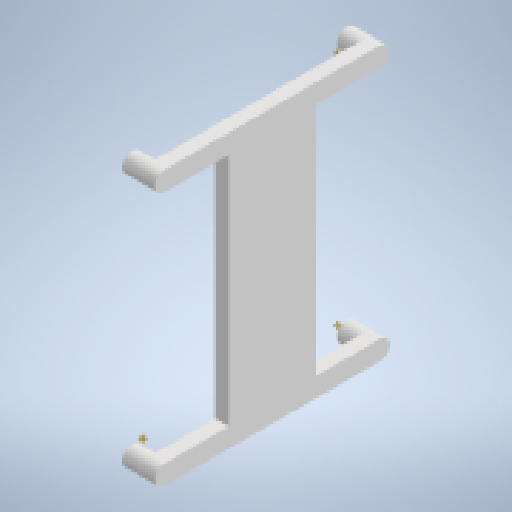
# Autodesk Inventor part: base
Saved by Autodesk Inventor 2025.2 (Build 292293000, 293)
## iProperties
Created: 2025-02-22
Part Number: base
Material: Générique
Document SubType Name: Modeling
Designer: antoi
Density: 1 g/cm^3
Appearance: Par défaut
Author: antoi
Autodesk Inventor part; units mm, degrees
ref_plane "YZ Plane" through (0, 0, 0) normal (1, 0, 0) x (0, 1, 0)
ref_plane "XZ Plane" through (0, 0, 0) normal (0, 1, 0) x (-1, 0, 0)
ref_plane "XY Plane" through (0, 0, 0) normal (0, 0, 1) x (1, 0, 0)
sketch "Esquisse1" plane through (0, 0, 0) normal (1, 0, 0) x (0, 1, 0)
  line L0 (7.5, 0) -> (138.9, 0)
  line L1 (146.4, -7.5) -> (146.4, -122.5)
  line L2 (138.9, -130) -> (7.5, -130)
  line L3 (0, -122.5) -> (0, -7.5)
  arc A0 (138.9, -130) -> (146.4, -122.5) centre (138.9, -122.5) ccw
  arc A1 (0, -122.5) -> (7.5, -130) centre (7.5, -122.5) ccw
  arc A2 (7.5, 0) -> (0, -7.5) centre (7.5, -7.5) ccw
  arc A3 (146.4, -7.5) -> (138.9, 0) centre (138.9, -7.5) ccw
  line L4 (15, -42.5) -> (131.4, -42.5)
  line L5 (131.4, -42.5) -> (131.4, -87.5)
  line L6 (131.4, -87.5) -> (15, -87.5)
  line L7 (15, -87.5) -> (15, -42.5)
  circle A4 centre (138.9, -122.5) radius 7.5
  line L8 (15, -42.5) -> (15, 0)
  line L9 (15, -87.5) -> (15, -130)
  line L10 (131.4, -87.5) -> (131.4, -130)
  line L11 (131.4, -42.5) -> (131.4, 0)
  circle A5 centre (7.5, -122.5) radius 7.5
  circle A6 centre (138.9, -7.5) radius 7.5
  circle A7 centre (7.5, -7.5) radius 7.5
  point P0 (0, 0)
  point P1 (146.4, -130)
  point P2 (146.4, 0)
  point P3 (0, -130)
  point P4 (73.2, -87.5)
  dimension "d0" = 146.4
  dimension "d1" = 130
  dimension "d2" = 7.5
  dimension "d3" = 7.5
  dimension "d4" = 116.4
  dimension "d5" = 45
  dimension "d11" = 42.5
  dimension "d12" = 42.5
  dimension "d13" = 15
  dimension "d104" = 131.4
  dimension "d107" = 115
  constraints: 24 end point, 14 point on line, 8 centre point, 8 point on circle, 8 tangent, 4 parallel, 4 perpendicular, 3 equal radius, 3 horizontal, 1 coincident, 1 midpoint, 1 vertical, 6 other
  measures "d0" distance of point (146.4, -130) point (0, -130)
  measures "d1" distance of point (146.4, 0) point (146.4, -130)
  measures "d2" radius of A0
  measures "d3" radius of A1
  measures "d4" distance of L5.end L6.end
  measures "d5" distance of L4.end L5.end
  measures "d11" distance between parallel lines of L0 L4
  measures "d12" distance from line of L2 point (73.2, -87.5)
  measures "d13" distance between parallel lines of L1 L10
  measures "d104" distance of A4.centre A5.centre
  measures "d107" distance of A4.centre A6.centre
sketch "Esquisse1 outline for Extrusion1" plane through (0, 0, 0) normal (1, 0, 0) x (0, 1, 0)
  line L0 (15, -87.5) -> (131.4, -87.5)
  line L1 (15, -130) -> (15, -87.5)
  line L2 (7.5, -130) -> (15, -130)
  arc A0 (0, -122.5) -> (7.5, -130) centre (7.5, -122.5) ccw
  line L3 (0, -7.5) -> (0, -122.5)
  arc A1 (7.5, 0) -> (0, -7.5) centre (7.5, -7.5) ccw
  line L4 (15, 0) -> (7.5, 0)
  line L5 (15, -42.5) -> (15, 0)
  line L6 (131.4, -42.5) -> (15, -42.5)
  line L7 (131.4, 0) -> (131.4, -42.5)
  line L8 (138.9, 0) -> (131.4, 0)
  arc A2 (146.4, -7.5) -> (138.9, 0) centre (138.9, -7.5) ccw
  line L9 (146.4, -122.5) -> (146.4, -7.5)
  arc A3 (138.9, -130) -> (146.4, -122.5) centre (138.9, -122.5) ccw
  line L10 (131.4, -130) -> (138.9, -130)
  line L11 (131.4, -87.5) -> (131.4, -130)
extrude "Extrusion1" add sketch "Esquisse1 outline for Extrusion1" along normal blind 7
sketch "Esquisse2" plane through (0, 0, 0) normal (-1, 0, 0) x (0, 0, 1)
  line L0 (-46.71, 27.48) -> (-83.29, 27.48)
  line L1 (-83.29, 27.48) -> (-83.29, 70.66)
  line L2 (-83.29, 70.66) -> (-46.71, 70.66)
  line L3 (-46.71, 70.66) -> (-46.71, 27.48)
  line L4 (-46.71, 75.74) -> (-83.29, 75.74)
  line L5 (-83.29, 75.74) -> (-83.29, 118.92)
  line L6 (-83.29, 118.92) -> (-46.71, 118.92)
  line L7 (-46.71, 118.92) -> (-46.71, 75.74)
  line L8 (-42.5, 131.4) -> (-42.5, 15) projected
  line L9 (-87.5, 15) -> (-87.5, 131.4) projected
  circle A0 centre (-83.29, 27.48) radius 2.3
  circle A1 centre (-46.71, 27.48) radius 2.3
  circle A2 centre (-46.71, 70.66) radius 2.3
  circle A3 centre (-83.29, 70.66) radius 2.3
  circle A4 centre (-83.29, 75.74) radius 2.3
  circle A5 centre (-46.71, 75.74) radius 2.3
  circle A6 centre (-46.71, 118.92) radius 2.3
  circle A7 centre (-83.29, 118.92) radius 2.3
  line L10 (-7.5, 0) -> (-122.5, 0) projected
  line L11 (-122.5, 146.4) -> (-7.5, 146.4) projected
  point P0 (0, 0)
  point P1 (-83.29, 49.07)
  dimension "d8" = 36.58
  dimension "d9" = 43.18
  dimension "d10" = 43.18
  dimension "d14" = 4.21
  dimension "d15" = 4.21
  dimension "d16" = 5.08
  dimension "d17" = 4.6
  dimension "d18" = 4.6
  dimension "d19" = 4.6
  dimension "d20" = 4.6
  dimension "d21" = 4.6
  dimension "d22" = 4.6
  dimension "d23" = 4.6
  dimension "d24" = 4.6
  dimension "d110" = 27.48
  dimension "d111" = 27.48
  constraints: 16 end point, 8 centre point, 8 coincident, 4 parallel, 2 horizontal, 2 perpendicular, 1 midpoint, 1 point on line
  measures "d8" distance of L1.end L2.end
  measures "d9" distance of L0.end L1.end
  measures "d10" distance of L4.end L5.end
  measures "d14" distance between parallel lines of L8 L3
  measures "d15" distance from line of L9 point (-83.29, 49.07)
  measures "d16" distance between parallel lines of L2 L4
  measures "d17" diameter of A0
  measures "d18" diameter of A1
  measures "d19" diameter of A2
  measures "d20" diameter of A3
  measures "d21" diameter of A4
  measures "d22" diameter of A5
  measures "d23" diameter of A6
  measures "d24" diameter of A7
  measures "d110" distance between parallel lines of L0 L10
  measures "d111" distance between parallel lines of L11 L6
sketch "Esquisse2 outline for Extrusion2" plane through (0, 0, 0) normal (-1, 0, 0) x (0, 0, 1)
  circle A0 centre (-46.71, 118.92) radius 2.3
  circle A1 centre (-83.29, 118.92) radius 2.3
  circle A2 centre (-83.29, 75.74) radius 2.3
  circle A3 centre (-46.71, 75.74) radius 2.3
  circle A4 centre (-83.29, 70.66) radius 2.3
  circle A5 centre (-46.71, 70.66) radius 2.3
  circle A6 centre (-46.71, 27.48) radius 2.3
  circle A7 centre (-83.29, 27.48) radius 2.3
extrude "Extrusion2" cut sketch "Esquisse2 outline for Extrusion2" against normal blind 5.7
sketch "Esquisse3" plane through (0, 0, 0) normal (-1, 0, 0) x (0, 0, 1)
  arc A0 (-7.5, 0) -> (0, 7.5) centre (-7.5, 7.5) ccw projected
  circle A1 centre (-7.5, 7.5) radius 7.5
  arc A2 (-130, 7.5) -> (-122.5, 0) centre (-122.5, 7.5) ccw projected
  circle A3 centre (-122.5, 7.5) radius 7.5
  arc A4 (-122.5, 146.4) -> (-130, 138.9) centre (-122.5, 138.9) ccw projected
  circle A5 centre (-122.5, 138.9) radius 7.5
  arc A6 (0, 138.9) -> (-7.5, 146.4) centre (-7.5, 138.9) ccw projected
  circle A7 centre (-7.5, 138.9) radius 7.5
  point P0 (0, 0)
  point P1 (-7.5, 0)
  point P2 (-7.5, 146.4)
  point P3 (-130, 7.5)
  constraints: 4 centre point, 4 coincident
sketch "Esquisse3 outline for Extrusion3" plane through (0, 0, 0) normal (-1, 0, 0) x (0, 0, 1)
  circle A0 centre (-7.5, 7.5) radius 7.5
  circle A1 centre (-7.5, 138.9) radius 7.5
  circle A2 centre (-122.5, 7.5) radius 7.5
  circle A3 centre (-122.5, 138.9) radius 7.5
extrude "Extrusion3" add sketch "Esquisse3 outline for Extrusion3" along normal blind 10
fillet "Congé1" radius 7.5 4 edges at (3.5, 131.4, 0) (3.5, 15, 0) (3.5, 131.4, -130) (3.5, 15, -130)
hole "Perçage5" at (-10, 7.5, -7.5) direction (1, 0, 0) diameter 6.3 depth 10
hole "Perçage6" at (-10, 138.9, -7.5) direction (1, 0, 0) diameter 6.3 depth 10
hole "Perçage7" at (-10, 138.9, -122.5) direction (1, 0, 0) diameter 6.3 depth 10
hole "Perçage8" at (-10, 7.5, -122.5) direction (1, 0, 0) diameter 6.3 depth 10
